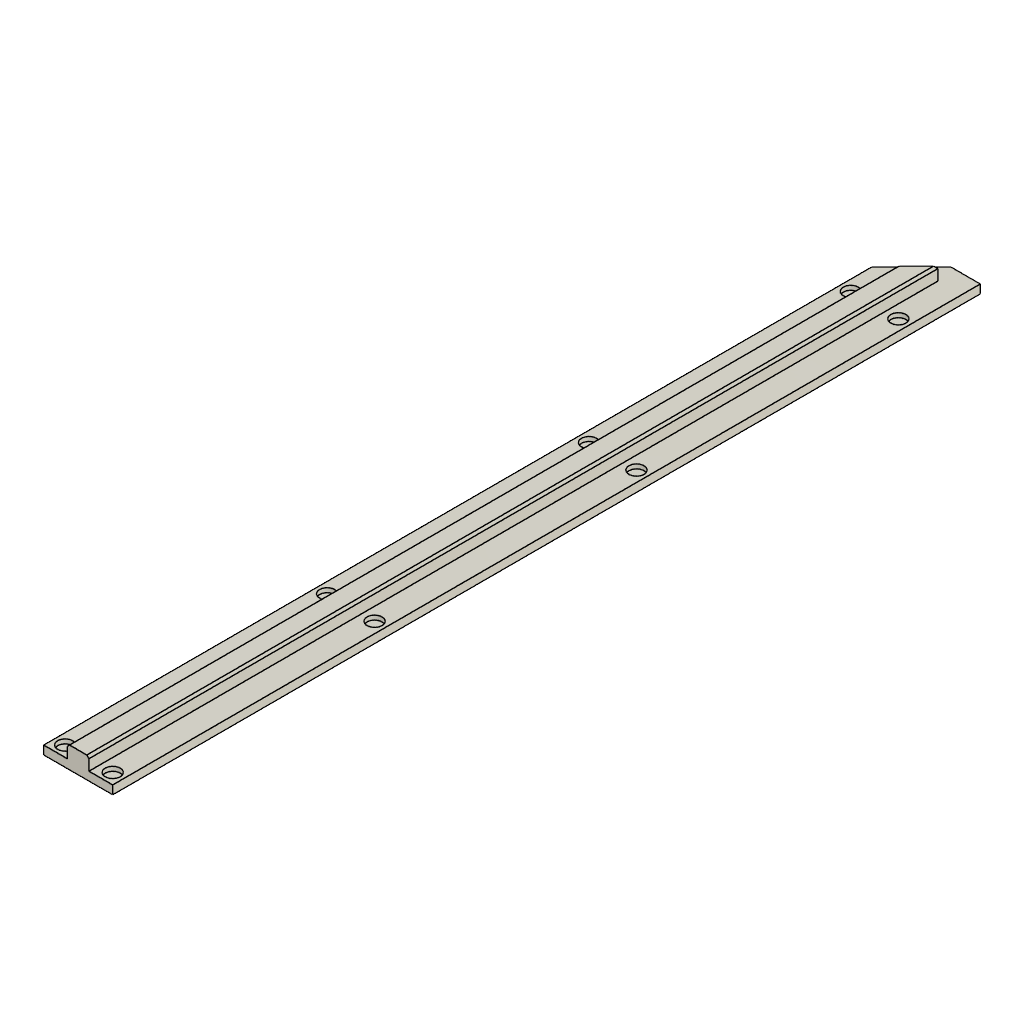
arcade_buttons_conduit_top (Autodesk Fusion 360 design; units mm, degrees)
part number: 2026-09-19-15-15-46-900
Autodesk Fusion 360 part; units mm, degrees
sketch "3D-printed conduit top outline" plane through (0, 0, 0) normal (0, 1, 0) x (1, 0, 0)
  line L0 (0, 0) -> (16, 0)
  line L1 (16, 0) -> (16, -2)
  line L2 (16, -2) -> (0, -2)
  line L3 (0, -2) -> (0, 0)
  dimension "d7" = 16
  dimension "d8" = 2
  constraint horizontal L0
  constraint vertical L1
  constraint horizontal L2
  constraint vertical L3
  constraint coincident L0.start L3.end
  measures "d7" distance of L0.start L0.end
  measures "d8" distance of L0.start L2.end
extrude "Extrude1" add sketch "3D-printed conduit top outline" along normal blind 201
sketch "Magnet holes" plane through (0, 0, 2) normal (0, 0, 1) x (-1, 0, 0)
  line L0 (0, 0) -> (-16, 0)
  line L1 (-16, 0) -> (-16, -201)
  line L2 (-16, -201) -> (0, -201)
  line L3 (0, -201) -> (0, 0)
  circle A0 centre (-2.5, -2.5) radius 2.5
  circle A1 centre (-13.5, -2.5) radius 2.5
  circle A2 centre (-2.5, -2.5) radius 1.75
  circle A3 centre (-13.5, -2.5) radius 1.75
  circle A4 centre (-2.5, -63.1667) radius 1.75
  circle A5 centre (-2.5, -63.1667) radius 2.5
  circle A6 centre (-13.5, -63.1667) radius 2.5
  circle A7 centre (-13.5, -63.1667) radius 1.75
  circle A8 centre (-2.5, -123.8333) radius 1.75
  circle A9 centre (-2.5, -123.8333) radius 2.5
  circle A10 centre (-13.5, -123.8333) radius 2.5
  circle A11 centre (-13.5, -123.8333) radius 1.75
  circle A12 centre (-2.5, -184.5) radius 1.75
  circle A13 centre (-2.5, -184.5) radius 2.5
  circle A14 centre (-13.5, -184.5) radius 2.5
  circle A15 centre (-13.5, -184.5) radius 1.75
  dimension "d11" = 5
  dimension "d12" = 5
  dimension "d13" = 3.5
  dimension "d14" = 3.5
  dimension "d17" = 0
  dimension "d18" = -182
  constraint concentric A0 A2
  constraint concentric A1 A3
  constraint tangent L3 A0
  constraint tangent L0 A0
  constraint tangent L1 A1
  constraint tangent L0 A1
  measures "d11" diameter of A0
  measures "d12" diameter of A1
  measures "d13" diameter of A2
  measures "d14" diameter of A3
extrude "Extrude2" cut sketch "Magnet holes" against normal blind 1 contours A2 | A3 | A4 | A7 | A8 | A11 | A12 | A15
sketch "Support rib" plane through (0, 0, 2) normal (0, 0, 1) x (-1, 0, 0)
  line L0 (0, 0) -> (-16, 0)
  line L1 (-16, 0) -> (-16, -201)
  line L2 (-16, -201) -> (0, -201)
  line L3 (0, -201) -> (0, 0)
  circle A0 centre (-13.5, -184.5) radius 1.75
  circle A1 centre (-13.5, -63.1667) radius 1.75
  circle A2 centre (-2.5, -2.5) radius 1.75
  circle A3 centre (-2.5, -123.8333) radius 1.75
  circle A4 centre (-2.5, -184.5) radius 1.75
  circle A5 centre (-2.5, -63.1667) radius 1.75
  circle A6 centre (-13.5, -2.5) radius 1.75
  circle A7 centre (-13.5, -123.8333) radius 1.75
  line L4 (-5.5, 0) -> (-10.5, 0)
  line L5 (-10.5, 0) -> (-10.5, -201)
  line L6 (-10.5, -201) -> (-5.5, -201)
  line L7 (-5.5, -201) -> (-5.5, 0)
  dimension "d23" = 5
  dimension "d24" = 5.5
  dimension "d25" = 5.5
  constraint horizontal L4
  constraint vertical L5
  constraint horizontal L6
  constraint vertical L7
  constraint coincident L2 L5.end
  constraint coincident L0 L4.start
  measures "d23" distance of L5 L7
  measures "d24" distance of L3 L7
  measures "d25" distance of L1 L5
extrude "Extrude3" add sketch "Support rib" along normal blind 3 contours L0 L2 L4 L5 L6 L7
chamfer "Chamfer1" distance 0.5 angle 45 2 edges at (5.5, 100.5, 5) (10.5, 100.5, 5)
sketch "End chamfer" plane through (0, 0, 2) normal (0, 0, 1) x (-1, 0, 0)
  line L0 (-10.5, -201) -> (-10.5, 0)
  line L1 (-10.5, 0) -> (-16, 0)
  line L2 (-16, 0) -> (-16, -201)
  line L3 (-16, -201) -> (-10.5, -201)
  circle A0 centre (-13.5, -123.8333) radius 1.75
  circle A1 centre (-13.5, -2.5) radius 1.75
  circle A2 centre (-13.5, -63.1667) radius 1.75
  circle A3 centre (-13.5, -184.5) radius 1.75
  line L4 (0, -191.828) -> (-9.172, -201)
  line L5 (0, 0) -> (0, -201)
  line L6 (-14.8289, -201) -> (0, -186.1711)
  line L7 (0, -191.828) -> (0, -201)
  line L8 (0, -201) -> (-9.172, -201)
  line L9 (-9.172, -201) -> (-14.8289, -201)
  line L10 (0, -191.828) -> (0, -186.1711)
  dimension "d30" = 6.828
  dimension "d31" = 135
  dimension "d32" = 4
  constraint coincident L3 L4.end
  constraint coincident L4.start L5
  constraint coincident L3 L6.start
  constraint coincident L5 L6.end
  constraint parallel L4 L6
  constraint coincident L5.end L7.end
  measures "d30" distance of L2.end L4.end
  measures "d31" angle of L3 L4
  measures "d32" distance of L4 L6
extrude "Extrude4" cut sketch "End chamfer" along normal blind 3 and the other way blind 2 contours L4 L5 L7 L8
extrude "Extrude5" cut sketch "End chamfer" along normal blind 3 contours L0 L3 L6 L9 | L0 L4 L5 L6 L9 L10
equation "conduit_length = 201 mm"
equation "conduit_width = 16 mm"
equation "conduit_wall_thickness = 2 mm"
equation "magnet_diameter = 3 mm"
equation "magnet_height = 1 mm"
equation "number_of_magnets_on_a_side = 4"
equation "d7 = conduit_width"
equation "d8 = conduit_wall_thickness"
equation "d9 = conduit_length"
equation "d11 = magnet_diameter + 2 mm"
equation "d12 = magnet_diameter + 2 mm"
equation "d13 = magnet_diameter + 0.5 mm"
equation "d14 = magnet_diameter + 0.5 mm"
equation "d16 = number_of_magnets_on_a_side"
equation "d18 = -conduit_length + ( magnet_diameter + 2 mm ) + 14 mm"
equation "d19 = -magnet_height"
equation "rib_width = 5 mm"
equation "rib_height = 3 mm"
equation "d23 = rib_width"
equation "d24 = ( conduit_width - rib_width ) / 2"
equation "d26 = rib_height"
equation "rib_chamfer = 0.5 mm"
equation "d29 = rib_chamfer"
equation "d32 = 2 * conduit_wall_thickness"
equation "d33 = rib_height"
equation "d35 = conduit_wall_thickness"
equation "d37 = rib_height"
named bodies: "Arcade buttons conduit top"
